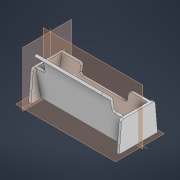
# Autodesk Inventor part: business card holder lgcc
Saved by Autodesk Inventor 2021 (Build 250183000, 183)
## iProperties
Created: 2020-08-19
Part Number: business card holder lgcc
Material: Generic
Document SubType Name: Modeling
Designer: brand
Density: 1 g/cm^3
Appearance: Default
Author: brand
Autodesk Inventor part; units mm, degrees
(part 1 of 6)
sketch "Block1" plane through (0, 0, 0) normal (0, 0, 1) x (1, 0, 0)
  line L0 (3.2262, -16.0033) -> (3.2322, -15.9973)
  spline S0 degree 3 poles (3.2322, -15.9973) (3.2262, -15.9973) (3.2262, -16.0033) (3.2262, -16.0033) knots 1 1 1 1 2 2 2 2
  line L1 (3.2322, -15.9973) -> (3.2262, -15.9973) construction
  line L2 (3.2262, -15.9973) -> (3.2262, -16.0033) construction
  line L3 (3.2262, -16.0033) -> (3.2262, -16.0033) construction
  line L4 (38.8954, -13.7894) -> (38.8894, -13.8014)
  spline S1 degree 3 poles (38.8894, -13.8014) (38.8895, -13.8014) (38.8954, -13.7954) (38.8954, -13.7894) knots 1 1 1 1 2 2 2 2
  line L5 (38.8894, -13.8014) -> (38.8894, -13.8014) construction
  line L6 (38.8894, -13.8014) -> (38.8954, -13.7954) construction
  line L7 (38.8954, -13.7954) -> (38.8954, -13.7894) construction
  spline S2 degree 3 poles (38.8894, -13.8014) (38.8835, -13.8074) (38.8774, -13.8134) (38.8774, -13.8194) knots 0 0 0 0 1 1 1 1
  line L8 (38.8894, -13.8014) -> (38.8835, -13.8074) construction
  line L9 (38.8835, -13.8074) -> (38.8774, -13.8134) construction
  line L10 (38.8774, -13.8134) -> (38.8774, -13.8194) construction
  spline S3 degree 3 poles (38.8774, -13.8194) (38.8774, -13.8194) (38.8835, -13.8134) (38.8894, -13.8014) knots 1 1 1 1 2 2 2 2
  line L11 (38.8774, -13.8194) -> (38.8774, -13.8194) construction
  line L12 (38.8774, -13.8194) -> (38.8835, -13.8134) construction
  line L13 (38.8835, -13.8134) -> (38.8894, -13.8014) construction
  spline S4 degree 3 poles (51.5732, -15.5233) (51.5732, -15.4813) (51.6092, -15.4273) (51.5732, -15.3793) (51.5432, -15.3433) (51.5432, -15.3673) (51.5132, -15.3613) (51.3932, -15.3133) (51.2792, -15.3433) (51.1712, -15.3973) (51.0332, -15.4693) (50.8112, -15.7153) (50.8952, -15.8953) (50.9192, -15.9433) (51.0272, -16.0393) (51.0692, -16.0573) (51.1832, -16.1173) (51.2432, -16.0393) (51.3152, -15.9733) (51.3992, -15.8953) (51.4592, -15.8653) (51.5012, -15.7693) (51.5132, -15.7453) (51.6572, -15.5233) (51.5732, -15.5233) knots 0 0 0 0 1 1 1 2 2 2 3 3 3 4 4 4 5 5 5 6 6 6 7 7 7 8 8 8 8
  line L14 (51.5732, -15.5233) -> (51.5732, -15.4813) construction
  line L15 (51.5732, -15.4813) -> (51.6092, -15.4273) construction
  line L16 (51.6092, -15.4273) -> (51.5732, -15.3793) construction
  line L17 (51.5732, -15.3793) -> (51.5432, -15.3433) construction
  line L18 (51.5432, -15.3433) -> (51.5432, -15.3673) construction
  line L19 (51.5432, -15.3673) -> (51.5132, -15.3613) construction
  line L20 (51.5132, -15.3613) -> (51.3932, -15.3133) construction
  line L21 (51.3932, -15.3133) -> (51.2792, -15.3433) construction
  line L22 (51.2792, -15.3433) -> (51.1712, -15.3973) construction
  line L23 (51.1712, -15.3973) -> (51.0332, -15.4693) construction
  line L24 (51.0332, -15.4693) -> (50.8112, -15.7153) construction
  line L25 (50.8112, -15.7153) -> (50.8952, -15.8953) construction
  line L26 (50.8952, -15.8953) -> (50.9192, -15.9433) construction
  line L27 (50.9192, -15.9433) -> (51.0272, -16.0393) construction
  line L28 (51.0272, -16.0393) -> (51.0692, -16.0573) construction
  line L29 (51.0692, -16.0573) -> (51.1832, -16.1173) construction
  line L30 (51.1832, -16.1173) -> (51.2432, -16.0393) construction
  line L31 (51.2432, -16.0393) -> (51.3152, -15.9733) construction
  line L32 (51.3152, -15.9733) -> (51.3992, -15.8953) construction
  line L33 (51.3992, -15.8953) -> (51.4592, -15.8653) construction
  line L34 (51.4592, -15.8653) -> (51.5012, -15.7693) construction
  line L35 (51.5012, -15.7693) -> (51.5132, -15.7453) construction
  line L36 (51.5132, -15.7453) -> (51.6572, -15.5233) construction
  line L37 (51.6572, -15.5233) -> (51.5732, -15.5233) construction
  spline S5 degree 3 poles (51.0512, -14.0894) (51.0512, -14.0894) (51.0572, -14.0954) (51.0512, -14.0834) knots 0 0 0 0 1 1 1 1
  line L38 (51.0512, -14.0894) -> (51.0512, -14.0894) construction
  line L39 (51.0512, -14.0894) -> (51.0572, -14.0954) construction
  line L40 (51.0572, -14.0954) -> (51.0512, -14.0834) construction
  spline S6 degree 3 poles (51.0512, -14.0834) (51.0212, -14.0414) (50.9792, -14.0714) (50.9372, -14.0834) knots 1 1 1 1 2 2 2 2
  line L41 (51.0512, -14.0834) -> (51.0212, -14.0414) construction
  line L42 (51.0212, -14.0414) -> (50.9792, -14.0714) construction
  line L43 (50.9792, -14.0714) -> (50.9372, -14.0834) construction
  spline S7 degree 3 poles (50.9372, -14.0834) (50.7632, -14.1194) (50.5832, -14.1614) (50.4032, -14.1914) knots 2 2 2 2 3 3 3 3
  line L44 (50.9372, -14.0834) -> (50.7632, -14.1194) construction
  line L45 (50.7632, -14.1194) -> (50.5832, -14.1614) construction
  line L46 (50.5832, -14.1614) -> (50.4032, -14.1914) construction
  spline S8 degree 3 poles (50.4032, -14.1914) (50.4692, -13.9754) (50.5352, -13.7474) (50.5592, -13.5254) knots 3 3 3 3 4 4 4 4
  line L47 (50.4032, -14.1914) -> (50.4692, -13.9754) construction
  line L48 (50.4692, -13.9754) -> (50.5352, -13.7474) construction
  line L49 (50.5352, -13.7474) -> (50.5592, -13.5254) construction
  spline S9 degree 3 poles (50.5592, -13.5254) (50.5712, -13.4414) (50.5772, -13.3514) (50.5592, -13.2674) knots 4 4 4 4 5 5 5 5
  line L50 (50.5592, -13.5254) -> (50.5712, -13.4414) construction
  line L51 (50.5712, -13.4414) -> (50.5772, -13.3514) construction
  line L52 (50.5772, -13.3514) -> (50.5592, -13.2674) construction
  spline S10 degree 3 poles (50.5592, -13.2674) (50.5472, -13.2134) (50.5292, -13.1594) (50.4992, -13.1114) knots 5 5 5 5 6 6 6 6
  line L53 (50.5592, -13.2674) -> (50.5472, -13.2134) construction
  line L54 (50.5472, -13.2134) -> (50.5292, -13.1594) construction
  line L55 (50.5292, -13.1594) -> (50.4992, -13.1114) construction
  spline S11 degree 3 poles (50.4992, -13.1114) (50.4992, -13.1113) (50.4272, -13.0214) (50.4452, -13.0694) knots 6 6 6 6 7 7 7 7
  line L56 (50.4992, -13.1114) -> (50.4992, -13.1114) construction
  line L57 (50.4992, -13.1114) -> (50.4272, -13.0214) construction
  line L58 (50.4272, -13.0214) -> (50.4452, -13.0694) construction
  line L59 (50.4452, -13.0694) -> (50.4392, -13.0634)
  line L60 (50.4392, -13.0634) -> (50.4152, -13.0154)
  line L61 (50.4152, -13.0154) -> (50.4392, -13.0394)
  spline S12 degree 3 poles (50.4392, -13.0394) (50.4452, -13.0034) (50.3433, -12.9374) (50.3432, -12.9374) knots 10 10 10 10 11 11 11 11
  line L62 (50.4392, -13.0394) -> (50.4452, -13.0034) construction
  line L63 (50.4452, -13.0034) -> (50.3432, -12.9374) construction
  line L64 (50.3432, -12.9374) -> (50.3432, -12.9374) construction
  spline S13 degree 3 poles (50.3432, -12.9374) (50.1932, -12.7874) (49.9892, -12.6734) (49.7852, -12.7874) knots 11 11 11 11 12 12 12 12
  line L65 (50.3432, -12.9374) -> (50.1932, -12.7874) construction
  line L66 (50.1932, -12.7874) -> (49.9892, -12.6734) construction
  line L67 (49.9892, -12.6734) -> (49.7852, -12.7874) construction
  spline S14 degree 3 poles (49.7852, -12.7874) (49.6592, -12.8594) (49.5573, -12.9794) (49.4732, -13.0994) knots 12 12 12 12 13 13 13 13
  line L68 (49.7852, -12.7874) -> (49.6592, -12.8594) construction
  line L69 (49.6592, -12.8594) -> (49.5573, -12.9794) construction
  line L70 (49.5573, -12.9794) -> (49.4732, -13.0994) construction
  spline S15 degree 3 poles (49.4732, -13.0994) (49.4432, -13.1414) (49.4132, -13.1894) (49.3892, -13.2374) knots 13 13 13 13 14 14 14 14
  line L71 (49.4732, -13.0994) -> (49.4432, -13.1414) construction
  line L72 (49.4432, -13.1414) -> (49.4132, -13.1894) construction
  line L73 (49.4132, -13.1894) -> (49.3892, -13.2374) construction
  spline S16 degree 3 poles (49.3892, -13.2374) (49.3652, -13.2854) (49.3292, -13.4414) (49.2933, -13.4654) knots 14 14 14 14 15 15 15 15
  line L74 (49.3892, -13.2374) -> (49.3652, -13.2854) construction
  line L75 (49.3652, -13.2854) -> (49.3292, -13.4414) construction
  line L76 (49.3292, -13.4414) -> (49.2933, -13.4654) construction
  spline S17 degree 3 poles (49.2933, -13.4654) (49.2632, -13.4894) (49.1733, -13.4954) (49.1312, -13.5194) knots 15 15 15 15 16 16 16 16
  line L77 (49.2933, -13.4654) -> (49.2632, -13.4894) construction
  line L78 (49.2632, -13.4894) -> (49.1733, -13.4954) construction
  line L79 (49.1733, -13.4954) -> (49.1312, -13.5194) construction
  spline S18 degree 3 poles (49.1312, -13.5194) (49.0712, -13.5434) (49.0173, -13.5734) (48.9692, -13.6094) knots 16 16 16 16 17 17 17 17
  line L80 (49.1312, -13.5194) -> (49.0712, -13.5434) construction
  line L81 (49.0712, -13.5434) -> (49.0173, -13.5734) construction
  line L82 (49.0173, -13.5734) -> (48.9692, -13.6094) construction
  spline S19 degree 3 poles (48.9692, -13.6094) (48.8553, -13.6814) (48.7653, -13.7834) (48.6812, -13.8854) knots 17 17 17 17 18 18 18 18
  line L83 (48.9692, -13.6094) -> (48.8553, -13.6814) construction
  line L84 (48.8553, -13.6814) -> (48.7653, -13.7834) construction
  line L85 (48.7653, -13.7834) -> (48.6812, -13.8854) construction
  spline S20 degree 3 poles (48.6812, -13.8854) (48.5373, -14.0774) (48.4653, -14.2934) (48.3632, -14.4854) knots 18 18 18 18 19 19 19 19
  line L86 (48.6812, -13.8854) -> (48.5373, -14.0774) construction
  line L87 (48.5373, -14.0774) -> (48.4653, -14.2934) construction
  line L88 (48.4653, -14.2934) -> (48.3632, -14.4854) construction
  spline S21 degree 3 poles (48.3632, -14.4854) (48.1713, -14.8513) (48.3813, -15.3313) (48.7353, -15.5053) knots 19 19 19 19 20 20 20 20
  line L89 (48.3632, -14.4854) -> (48.1713, -14.8513) construction
  line L90 (48.1713, -14.8513) -> (48.3813, -15.3313) construction
  line L91 (48.3813, -15.3313) -> (48.7353, -15.5053) construction
  spline S22 degree 3 poles (48.7353, -15.5053) (48.8492, -15.5593) (48.9812, -15.5833) (49.1012, -15.5713) knots 20 20 20 20 21 21 21 21
  line L92 (48.7353, -15.5053) -> (48.8492, -15.5593) construction
  line L93 (48.8492, -15.5593) -> (48.9812, -15.5833) construction
  line L94 (48.9812, -15.5833) -> (49.1012, -15.5713) construction
  spline S23 degree 3 poles (49.1012, -15.5713) (49.2273, -15.5533) (49.3472, -15.4873) (49.4432, -15.4153) knots 21 21 21 21 22 22 22 22
  line L95 (49.1012, -15.5713) -> (49.2273, -15.5533) construction
  line L96 (49.2273, -15.5533) -> (49.3472, -15.4873) construction
  line L97 (49.3472, -15.4873) -> (49.4432, -15.4153) construction
  spline S24 degree 3 poles (49.4432, -15.4153) (49.5332, -15.3493) (49.7312, -15.2293) (49.7672, -15.1273) knots 22 22 22 22 23 23 23 23
  line L98 (49.4432, -15.4153) -> (49.5332, -15.3493) construction
  line L99 (49.5332, -15.3493) -> (49.7312, -15.2293) construction
  line L100 (49.7312, -15.2293) -> (49.7672, -15.1273) construction
  spline S25 degree 3 poles (49.7672, -15.1273) (49.7672, -15.1213) (49.7552, -15.1273) (49.7372, -15.1453) knots 23 23 23 23 24 24 24 24
  line L101 (49.7672, -15.1273) -> (49.7672, -15.1213) construction
  line L102 (49.7672, -15.1213) -> (49.7552, -15.1273) construction
  line L103 (49.7552, -15.1273) -> (49.7372, -15.1453) construction
  line L104 (49.7372, -15.1453) -> (49.9112, -14.9413)
  spline S26 degree 3 poles (49.9112, -14.9413) (49.9172, -14.9473) (49.8693, -15.0073) (49.8692, -15.0073) knots 25 25 25 25 26 26 26 26
  line L105 (49.9112, -14.9413) -> (49.9172, -14.9473) construction
  line L106 (49.9172, -14.9473) -> (49.8692, -15.0073) construction
  line L107 (49.8692, -15.0073) -> (49.8692, -15.0073) construction
  spline S27 degree 3 poles (49.8692, -15.0073) (49.9112, -15.0253) (50.1272, -14.7074) (50.1512, -14.6833) knots 26 26 26 26 27 27 27 27
  line L108 (49.8692, -15.0073) -> (49.9112, -15.0253) construction
  line L109 (49.9112, -15.0253) -> (50.1272, -14.7074) construction
  line L110 (50.1272, -14.7074) -> (50.1512, -14.6833) construction
  spline S28 degree 3 poles (50.1512, -14.6833) (50.1932, -14.6113) (50.2352, -14.5333) (50.2832, -14.4614) knots 27 27 27 27 28 28 28 28
  line L111 (50.1512, -14.6833) -> (50.1932, -14.6113) construction
  line L112 (50.1932, -14.6113) -> (50.2352, -14.5333) construction
  line L113 (50.2352, -14.5333) -> (50.2832, -14.4614) construction
  spline S29 degree 3 poles (50.2832, -14.4614) (50.3252, -14.4073) (50.3132, -14.4134) (50.3732, -14.3894) knots 28 28 28 28 29 29 29 29
  line L114 (50.2832, -14.4614) -> (50.3252, -14.4073) construction
  line L115 (50.3252, -14.4073) -> (50.3132, -14.4134) construction
  line L116 (50.3132, -14.4134) -> (50.3732, -14.3894) construction
  spline S30 degree 3 poles (50.3732, -14.3894) (50.3672, -14.3954) (50.4452, -14.3714) (50.4572, -14.3714) knots 29 29 29 29 30 30 30 30
  line L117 (50.3732, -14.3894) -> (50.3672, -14.3954) construction
  line L118 (50.3672, -14.3954) -> (50.4452, -14.3714) construction
  line L119 (50.4452, -14.3714) -> (50.4572, -14.3714) construction
  spline S31 degree 3 poles (50.4572, -14.3714) (50.5232, -14.3594) (51.2252, -14.3114) (51.0512, -14.0894) knots 30 30 30 30 31 31 31 31
  line L120 (50.4572, -14.3714) -> (50.5232, -14.3594) construction
  line L121 (50.5232, -14.3594) -> (51.2252, -14.3114) construction
  line L122 (51.2252, -14.3114) -> (51.0512, -14.0894) construction
  spline S32 degree 3 poles (49.7492, -13.2434) (49.7492, -13.2494) (49.7433, -13.2494) (49.7432, -13.2494) knots 0 0 0 0 1 1 1 1
  line L123 (49.7492, -13.2434) -> (49.7492, -13.2494) construction
  line L124 (49.7492, -13.2494) -> (49.7432, -13.2494) construction
  line L125 (49.7432, -13.2494) -> (49.7432, -13.2494) construction
  line L126 (49.7432, -13.2494) -> (49.7492, -13.2434)
  line L127 (49.7492, -13.2434) -> (49.7432, -13.2494)
  spline S33 degree 3 poles (49.7432, -13.2494) (49.7433, -13.2494) (49.7492, -13.2494) (49.7492, -13.2434) knots 1 1 1 1 2 2 2 2
  line L128 (49.7432, -13.2494) -> (49.7432, -13.2494) construction
  line L129 (49.7432, -13.2494) -> (49.7492, -13.2494) construction
  line L130 (49.7492, -13.2494) -> (49.7492, -13.2434) construction
  spline S34 degree 3 poles (47.9672, -14.3534) (47.9012, -14.3474) (47.8532, -14.4914) (47.8292, -14.5273) knots 0 0 0 0 1 1 1 1
  line L131 (47.9672, -14.3534) -> (47.9012, -14.3474) construction
  line L132 (47.9012, -14.3474) -> (47.8532, -14.4914) construction
  line L133 (47.8532, -14.4914) -> (47.8292, -14.5273) construction
  spline S35 degree 3 poles (47.8292, -14.5273) (47.6493, -14.8214) (47.4392, -15.0974) (47.2052, -15.3493) knots 1 1 1 1 2 2 2 2
  line L134 (47.8292, -14.5273) -> (47.6493, -14.8214) construction
  line L135 (47.6493, -14.8214) -> (47.4392, -15.0974) construction
  line L136 (47.4392, -15.0974) -> (47.2052, -15.3493) construction
  spline S36 degree 3 poles (47.2052, -15.3493) (46.9653, -15.6133) (46.6652, -15.8953) (46.2993, -15.9793) knots 2 2 2 2 3 3 3 3
  line L137 (47.2052, -15.3493) -> (46.9653, -15.6133) construction
  line L138 (46.9653, -15.6133) -> (46.6652, -15.8953) construction
  line L139 (46.6652, -15.8953) -> (46.2993, -15.9793) construction
  spline S37 degree 3 poles (46.2993, -15.9793) (46.2513, -15.9913) (46.1973, -15.9973) (46.1433, -15.9973) knots 3 3 3 3 4 4 4 4
  line L140 (46.2993, -15.9793) -> (46.2513, -15.9913) construction
  line L141 (46.2513, -15.9913) -> (46.1973, -15.9973) construction
  line L142 (46.1973, -15.9973) -> (46.1433, -15.9973) construction
  spline S38 degree 3 poles (46.1433, -15.9973) (46.0712, -15.9913) (46.0052, -15.9733) (45.9513, -15.9193) knots 4 4 4 4 5 5 5 5
  line L143 (46.1433, -15.9973) -> (46.0712, -15.9913) construction
  line L144 (46.0712, -15.9913) -> (46.0052, -15.9733) construction
  line L145 (46.0052, -15.9733) -> (45.9513, -15.9193) construction
  spline S39 degree 3 poles (45.9513, -15.9193) (45.9213, -15.8893) (45.8913, -15.7873) (45.8553, -15.7693) knots 5 5 5 5 6 6 6 6
  line L146 (45.9513, -15.9193) -> (45.9213, -15.8893) construction
  line L147 (45.9213, -15.8893) -> (45.8913, -15.7873) construction
  line L148 (45.8913, -15.7873) -> (45.8553, -15.7693) construction
  spline S40 degree 3 poles (45.8553, -15.7693) (45.8553, -15.7393) (45.8493, -15.7093) (45.8433, -15.6913) knots 6 6 6 6 7 7 7 7
  line L149 (45.8553, -15.7693) -> (45.8553, -15.7393) construction
  line L150 (45.8553, -15.7393) -> (45.8493, -15.7093) construction
  line L151 (45.8493, -15.7093) -> (45.8433, -15.6913) construction
  line L152 (45.8433, -15.6913) -> (45.8351, -15.6553)
  spline S41 degree 3 poles (45.8351, -15.6553) (45.8291, -15.4753) (45.8333, -15.3073) (45.875, -15.1213) knots 8 8 8 8 9 9 9 9
  line L153 (45.8351, -15.6553) -> (45.8291, -15.4753) construction
  line L154 (45.8291, -15.4753) -> (45.8333, -15.3073) construction
  line L155 (45.8333, -15.3073) -> (45.875, -15.1213) construction
  line L156 (45.875, -15.1213) -> (45.875, -15.1153)
  spline S42 degree 3 poles (45.875, -15.1153) (45.875, -15.1101) (45.8724, -15.1089) (45.8717, -15.1049) knots 10 10 10 10 11 11 11 11
  line L157 (45.875, -15.1153) -> (45.875, -15.1101) construction
  line L158 (45.875, -15.1101) -> (45.8724, -15.1089) construction
  line L159 (45.8724, -15.1089) -> (45.8717, -15.1049) construction
  spline S43 degree 3 poles (45.8717, -15.1049) (45.8737, -15.1029) (45.875, -15.1011) (45.875, -15.0974) knots 11 11 11 11 12 12 12 12
  line L160 (45.8717, -15.1049) -> (45.8737, -15.1029) construction
  line L161 (45.8737, -15.1029) -> (45.875, -15.1011) construction
  line L162 (45.875, -15.1011) -> (45.875, -15.0974) construction
  line L163 (45.875, -15.0974) -> (45.875, -15.0673)
  spline S44 degree 3 poles (45.875, -15.0673) (45.9167, -14.7134) (46.0601, -14.3654) (46.1861, -14.0234) knots 13 13 13 13 14 14 14 14
  line L164 (45.875, -15.0673) -> (45.9167, -14.7134) construction
  line L165 (45.9167, -14.7134) -> (46.0601, -14.3654) construction
  line L166 (46.0601, -14.3654) -> (46.1861, -14.0234) construction
  spline S45 degree 3 poles (46.1861, -14.0234) (46.3181, -13.6634) (46.4407, -13.3094) (46.6087, -12.9674) knots 14 14 14 14 15 15 15 15
  line L167 (46.1861, -14.0234) -> (46.3181, -13.6634) construction
  line L168 (46.3181, -13.6634) -> (46.4407, -13.3094) construction
  line L169 (46.4407, -13.3094) -> (46.6087, -12.9674) construction
  spline S46 degree 3 poles (46.6087, -12.9674) (46.7647, -12.6434) (46.943, -12.3254) (47.147, -12.0314) knots 15 15 15 15 16 16 16 16
  line L170 (46.6087, -12.9674) -> (46.7647, -12.6434) construction
  line L171 (46.7647, -12.6434) -> (46.943, -12.3254) construction
  line L172 (46.943, -12.3254) -> (47.147, -12.0314) construction
  spline S47 degree 3 poles (47.147, -12.0314) (47.3269, -11.7614) (47.5421, -11.4674) (47.8181, -11.2874) knots 16 16 16 16 17 17 17 17
  line L173 (47.147, -12.0314) -> (47.3269, -11.7614) construction
  line L174 (47.3269, -11.7614) -> (47.5421, -11.4674) construction
  line L175 (47.5421, -11.4674) -> (47.8181, -11.2874) construction
  spline S48 degree 3 poles (47.8181, -11.2874) (47.9021, -11.2634) (47.9857, -11.1734) (48.0937, -11.1914) knots 17 17 17 17 18 18 18 18
  line L176 (47.8181, -11.2874) -> (47.9021, -11.2634) construction
  line L177 (47.9021, -11.2634) -> (47.9857, -11.1734) construction
  line L178 (47.9857, -11.1734) -> (48.0937, -11.1914) construction
  spline S49 degree 3 poles (48.0937, -11.1914) (48.2017, -11.2094) (48.2014, -11.3234) (48.1774, -11.4314) knots 18 18 18 18 19 19 19 19
  line L179 (48.0937, -11.1914) -> (48.2017, -11.2094) construction
  line L180 (48.2017, -11.2094) -> (48.2014, -11.3234) construction
  line L181 (48.2014, -11.3234) -> (48.1774, -11.4314) construction
  spline S50 degree 3 poles (48.1774, -11.4314) (48.2074, -11.3474) (48.2253, -11.2574) (48.1534, -11.1974) knots 19 19 19 19 20 20 20 20
  line L182 (48.1774, -11.4314) -> (48.2074, -11.3474) construction
  line L183 (48.2074, -11.3474) -> (48.2253, -11.2574) construction
  line L184 (48.2253, -11.2574) -> (48.1534, -11.1974) construction
  spline S51 degree 3 poles (48.1534, -11.1974) (48.0573, -11.1254) (47.8713, -11.2394) (47.7933, -11.2934) knots 20 20 20 20 21 21 21 21
  line L185 (48.1534, -11.1974) -> (48.0573, -11.1254) construction
  line L186 (48.0573, -11.1254) -> (47.8713, -11.2394) construction
  line L187 (47.8713, -11.2394) -> (47.7933, -11.2934) construction
  spline S52 degree 3 poles (47.7933, -11.2934) (47.7573, -11.3054) (47.7213, -11.3294) (47.6913, -11.3534) knots 21 21 21 21 22 22 22 22
  line L188 (47.7933, -11.2934) -> (47.7573, -11.3054) construction
  line L189 (47.7573, -11.3054) -> (47.7213, -11.3294) construction
  line L190 (47.7213, -11.3294) -> (47.6913, -11.3534) construction
  spline S53 degree 3 poles (47.6913, -11.3534) (47.7093, -11.3354) (47.7332, -11.3174) (47.7632, -11.2994) knots 22 22 22 22 23 23 23 23
  line L191 (47.6913, -11.3534) -> (47.7093, -11.3354) construction
  line L192 (47.7093, -11.3354) -> (47.7332, -11.3174) construction
  line L193 (47.7332, -11.3174) -> (47.7632, -11.2994) construction
  line L194 (47.7632, -11.2994) -> (47.7332, -11.3114)
  line L195 (47.7332, -11.3114) -> (47.8172, -11.2634)
  spline S54 degree 3 poles (47.8172, -11.2634) (47.9132, -11.2094) (48.1292, -11.0894) (48.2012, -11.2454) knots 25 25 25 25 26 26 26 26
  line L196 (47.8172, -11.2634) -> (47.9132, -11.2094) construction
  line L197 (47.9132, -11.2094) -> (48.1292, -11.0894) construction
  line L198 (48.1292, -11.0894) -> (48.2012, -11.2454) construction
  spline S55 degree 3 poles (48.2012, -11.2454) (48.2552, -11.3714) (48.1712, -11.5814) (48.1292, -11.7014) knots 26 26 26 26 27 27 27 27
  line L199 (48.2012, -11.2454) -> (48.2552, -11.3714) construction
  line L200 (48.2552, -11.3714) -> (48.1712, -11.5814) construction
  line L201 (48.1712, -11.5814) -> (48.1292, -11.7014) construction
  spline S56 degree 3 poles (48.1292, -11.7014) (48.0512, -11.9054) (47.9552, -12.0974) (47.8532, -12.2894) knots 27 27 27 27 28 28 28 28
  line L202 (48.1292, -11.7014) -> (48.0512, -11.9054) construction
  line L203 (48.0512, -11.9054) -> (47.9552, -12.0974) construction
  line L204 (47.9552, -12.0974) -> (47.8532, -12.2894) construction
  spline S57 degree 3 poles (47.8532, -12.2894) (47.8712, -12.2474) (47.9432, -12.0887) (47.9432, -12.0885) knots 28 28 28 28 29 29 29 29
  line L205 (47.8532, -12.2894) -> (47.8712, -12.2474) construction
  line L206 (47.8712, -12.2474) -> (47.9432, -12.0885) construction
  line L207 (47.9432, -12.0885) -> (47.9432, -12.0885) construction
  spline S58 degree 3 poles (47.9432, -12.0885) (47.9012, -12.0825) (47.7092, -12.5417) (47.6732, -12.5417) knots 29 29 29 29 30 30 30 30
  line L208 (47.9432, -12.0885) -> (47.9012, -12.0825) construction
  line L209 (47.9012, -12.0825) -> (47.7092, -12.5417) construction
  line L210 (47.7092, -12.5417) -> (47.6732, -12.5417) construction
  line L211 (47.6732, -12.5417) -> (47.6792, -12.5417)
  spline S59 degree 3 poles (47.6792, -12.5417) (47.6552, -12.5417) (47.6372, -12.5745) (47.6372, -12.5805) knots 31 31 31 31 32 32 32 32
  line L212 (47.6792, -12.5417) -> (47.6552, -12.5417) construction
  line L213 (47.6552, -12.5417) -> (47.6372, -12.5745) construction
  line L214 (47.6372, -12.5745) -> (47.6372, -12.5805) construction
  spline S60 degree 3 poles (47.6372, -12.5805) (47.6252, -12.6525) (47.7092, -12.633) (47.7572, -12.627) knots 32 32 32 32 33 33 33 33
  line L215 (47.6372, -12.5805) -> (47.6252, -12.6525) construction
  line L216 (47.6252, -12.6525) -> (47.7092, -12.633) construction
  line L217 (47.7092, -12.633) -> (47.7572, -12.627) construction
  spline S61 degree 3 poles (47.7572, -12.627) (47.9612, -12.603) (48.2184, -12.4282) (48.3504, -12.2782) knots 33 33 33 33 34 34 34 34
  line L218 (47.7572, -12.627) -> (47.9612, -12.603) construction
  line L219 (47.9612, -12.603) -> (48.2184, -12.4282) construction
  line L220 (48.2184, -12.4282) -> (48.3504, -12.2782) construction
  spline S62 degree 3 poles (48.3504, -12.2782) (48.4945, -12.1162) (48.5417, -11.8694) (48.5417, -11.6534) knots 34 34 34 34 35 35 35 35
  line L221 (48.3504, -12.2782) -> (48.4945, -12.1162) construction
  line L222 (48.4945, -12.1162) -> (48.5417, -11.8694) construction
  line L223 (48.5417, -11.8694) -> (48.5417, -11.6534) construction
  line L224 (48.5417, -11.6534) -> (48.5417, -11.6474)
  spline S63 degree 3 poles (48.5417, -11.6474) (48.5417, -11.2394) (48.2604, -10.7234) (47.7745, -10.7534) knots 36 36 36 36 37 37 37 37
  line L225 (48.5417, -11.6474) -> (48.5417, -11.2394) construction
  line L226 (48.5417, -11.2394) -> (48.2604, -10.7234) construction
  line L227 (48.2604, -10.7234) -> (47.7745, -10.7534) construction
  spline S64 degree 3 poles (47.7745, -10.7534) (47.5045, -10.7654) (47.2559, -11.0294) (47.0819, -11.2094) knots 37 37 37 37 38 38 38 38
  line L228 (47.7745, -10.7534) -> (47.5045, -10.7654) construction
  line L229 (47.5045, -10.7654) -> (47.2559, -11.0294) construction
  line L230 (47.2559, -11.0294) -> (47.0819, -11.2094) construction
  spline S65 degree 3 poles (47.0819, -11.2094) (46.9559, -11.3534) (46.8375, -11.5094) (46.7295, -11.6654) knots 38 38 38 38 39 39 39 39
  line L231 (47.0819, -11.2094) -> (46.9559, -11.3534) construction
  line L232 (46.9559, -11.3534) -> (46.8375, -11.5094) construction
  line L233 (46.8375, -11.5094) -> (46.7295, -11.6654) construction
  spline S66 degree 3 poles (46.7295, -11.6654) (46.6816, -11.7374) (46.6344, -11.8034) (46.5924, -11.8754) knots 39 39 39 39 40 40 40 40
  line L234 (46.7295, -11.6654) -> (46.6816, -11.7374) construction
  line L235 (46.6816, -11.7374) -> (46.6344, -11.8034) construction
  line L236 (46.6344, -11.8034) -> (46.5924, -11.8754) construction
  spline S67 degree 3 poles (46.5924, -11.8754) (46.5444, -11.9414) (46.4489, -12.0434) (46.4248, -12.1214) knots 40 40 40 40 41 41 41 41
  line L237 (46.5924, -11.8754) -> (46.5444, -11.9414) construction
  line L238 (46.5444, -11.9414) -> (46.4489, -12.0434) construction
  line L239 (46.4489, -12.0434) -> (46.4248, -12.1214) construction
  spline S68 degree 3 poles (46.4248, -12.1214) (46.4249, -12.1214) (46.455, -12.0854) (46.479, -12.0614) knots 41 41 41 41 42 42 42 42
  line L240 (46.4248, -12.1214) -> (46.4248, -12.1214) construction
  line L241 (46.4248, -12.1214) -> (46.455, -12.0854) construction
  line L242 (46.455, -12.0854) -> (46.479, -12.0614) construction
  spline S69 degree 3 poles (46.479, -12.0614) (46.413, -12.1634) (46.3531, -12.2714) (46.2931, -12.3734) knots 42 42 42 42 43 43 43 43
  line L243 (46.479, -12.0614) -> (46.413, -12.1634) construction
  line L244 (46.413, -12.1634) -> (46.3531, -12.2714) construction
  line L245 (46.3531, -12.2714) -> (46.2931, -12.3734) construction
  spline S70 degree 3 poles (46.2931, -12.3734) (46.2872, -12.3674) (46.3292, -12.2835) (46.3292, -12.2834) knots 43 43 43 43 44 44 44 44
  line L246 (46.2931, -12.3734) -> (46.2872, -12.3674) construction
  line L247 (46.2872, -12.3674) -> (46.3292, -12.2834) construction
  line L248 (46.3292, -12.2834) -> (46.3292, -12.2834) construction
  spline S71 degree 3 poles (46.3292, -12.2834) (46.2752, -12.2714) (46.0292, -12.7634) (45.9992, -12.8174) knots 44 44 44 44 45 45 45 45
  line L249 (46.3292, -12.2834) -> (46.2752, -12.2714) construction
  line L250 (46.2752, -12.2714) -> (46.0292, -12.7634) construction
  line L251 (46.0292, -12.7634) -> (45.9992, -12.8174) construction
  spline S72 degree 3 poles (45.9992, -12.8174) (45.8912, -13.0154) (45.7953, -13.2134) (45.7293, -13.4234) knots 45 45 45 45 46 46 46 46
  line L252 (45.9992, -12.8174) -> (45.8912, -13.0154) construction
  line L253 (45.8912, -13.0154) -> (45.7953, -13.2134) construction
  line L254 (45.7953, -13.2134) -> (45.7293, -13.4234) construction
  spline S73 degree 3 poles (45.7293, -13.4234) (45.6573, -13.6574) (45.5613, -13.8794) (45.4893, -14.1074) knots 46 46 46 46 47 47 47 47
  line L255 (45.7293, -13.4234) -> (45.6573, -13.6574) construction
  line L256 (45.6573, -13.6574) -> (45.5613, -13.8794) construction
  line L257 (45.5613, -13.8794) -> (45.4893, -14.1074) construction
  spline S74 degree 3 poles (45.4893, -14.1074) (45.4533, -14.2214) (45.4173, -14.3294) (45.3933, -14.4434) knots 47 47 47 47 48 48 48 48
  line L258 (45.4893, -14.1074) -> (45.4533, -14.2214) construction
  line L259 (45.4533, -14.2214) -> (45.4173, -14.3294) construction
  line L260 (45.4173, -14.3294) -> (45.3933, -14.4434) construction
  spline S75 degree 3 poles (45.3933, -14.4434) (45.3813, -14.4974) (45.3693, -14.5453) (45.3633, -14.5993) knots 48 48 48 48 49 49 49 49
  line L261 (45.3933, -14.4434) -> (45.3813, -14.4974) construction
  line L262 (45.3813, -14.4974) -> (45.3693, -14.5453) construction
  line L263 (45.3693, -14.5453) -> (45.3633, -14.5993) construction
  spline S76 degree 3 poles (45.3633, -14.5993) (45.3633, -14.6053) (45.3513, -14.7014) (45.3633, -14.6894) knots 49 49 49 49 50 50 50 50
  line L264 (45.3633, -14.5993) -> (45.3633, -14.6053) construction
  line L265 (45.3633, -14.6053) -> (45.3513, -14.7014) construction
  line L266 (45.3513, -14.7014) -> (45.3633, -14.6894) construction
  spline S77 degree 3 poles (45.3633, -14.6894) (45.3513, -14.7313) (45.3513, -14.7853) (45.3453, -14.8274) knots 50 50 50 50 51 51 51 51
  line L267 (45.3633, -14.6894) -> (45.3513, -14.7313) construction
  line L268 (45.3513, -14.7313) -> (45.3513, -14.7853) construction
  line L269 (45.3513, -14.7853) -> (45.3453, -14.8274) construction
  spline S78 degree 3 poles (45.3453, -14.8274) (45.3453, -14.8272) (45.3453, -14.7253) (45.3513, -14.7134) knots 51 51 51 51 52 52 52 52
  line L270 (45.3453, -14.8274) -> (45.3453, -14.8274) construction
  line L271 (45.3453, -14.8274) -> (45.3453, -14.7253) construction
  line L272 (45.3453, -14.7253) -> (45.3513, -14.7134) construction
  spline S79 degree 3 poles (45.3513, -14.7134) (45.3273, -14.7433) (45.3453, -14.8573) (45.3393, -14.8693) knots 52 52 52 52 53 53 53 53
  line L273 (45.3513, -14.7134) -> (45.3273, -14.7433) construction
  line L274 (45.3273, -14.7433) -> (45.3453, -14.8573) construction
  line L275 (45.3453, -14.8573) -> (45.3393, -14.8693) construction
  spline S80 degree 3 poles (45.3393, -14.8693) (45.3093, -15.0974) (45.2613, -15.3373) (45.3393, -15.5593) knots 53 53 53 53 54 54 54 54
  line L276 (45.3393, -14.8693) -> (45.3093, -15.0974) construction
  line L277 (45.3093, -15.0974) -> (45.2613, -15.3373) construction
  line L278 (45.2613, -15.3373) -> (45.3393, -15.5593) construction
  spline S81 degree 3 poles (45.3393, -15.5593) (45.4413, -15.8653) (45.6933, -16.1173) (45.9693, -16.2793) knots 54 54 54 54 55 55 55 55
  line L279 (45.3393, -15.5593) -> (45.4413, -15.8653) construction
  line L280 (45.4413, -15.8653) -> (45.6933, -16.1173) construction
  line L281 (45.6933, -16.1173) -> (45.9693, -16.2793) construction
  spline S82 degree 3 poles (45.9693, -16.2793) (46.1133, -16.3693) (46.3053, -16.4713) (46.4853, -16.4593) knots 55 55 55 55 56 56 56 56
  line L282 (45.9693, -16.2793) -> (46.1133, -16.3693) construction
  line L283 (46.1133, -16.3693) -> (46.3053, -16.4713) construction
  line L284 (46.3053, -16.4713) -> (46.4853, -16.4593) construction
  spline S83 degree 3 poles (46.4853, -16.4593) (46.6953, -16.4473) (46.8993, -16.2733) (47.0553, -16.1473) knots 56 56 56 56 57 57 57 57
  line L285 (46.4853, -16.4593) -> (46.6953, -16.4473) construction
  line L286 (46.6953, -16.4473) -> (46.8993, -16.2733) construction
  line L287 (46.8993, -16.2733) -> (47.0553, -16.1473) construction
  spline S84 degree 3 poles (47.0553, -16.1473) (47.5112, -15.7633) (47.9252, -15.2233) (48.0032, -14.6113) knots 57 57 57 57 58 58 58 58
  line L288 (47.0553, -16.1473) -> (47.5112, -15.7633) construction
  line L289 (47.5112, -15.7633) -> (47.9252, -15.2233) construction
  line L290 (47.9252, -15.2233) -> (48.0032, -14.6113) construction
  spline S85 degree 3 poles (48.0032, -14.6113) (48.0092, -14.5694) (48.0392, -14.3594) (47.9672, -14.3534) knots 58 58 58 58 59 59 59 59
  line L291 (48.0032, -14.6113) -> (48.0092, -14.5694) construction
  line L292 (48.0092, -14.5694) -> (48.0392, -14.3594) construction
  line L293 (48.0392, -14.3594) -> (47.9672, -14.3534) construction
  spline S86 degree 3 poles (48.1412, -11.5814) (48.1472, -11.5694) (48.1472, -11.5634) (48.1472, -11.5574) (48.1592, -11.5214) (48.1712, -11.4794) (48.1772, -11.4314) (48.1652, -11.4854) (48.1412, -11.5394) (48.1412, -11.5814) knots 0 0 0 0 1 1 1 2 2 2 3 3 3 3
  line L294 (48.1412, -11.5814) -> (48.1472, -11.5694) construction
  line L295 (48.1472, -11.5694) -> (48.1472, -11.5634) construction
  line L296 (48.1472, -11.5634) -> (48.1472, -11.5574) construction
  line L297 (48.1472, -11.5574) -> (48.1592, -11.5214) construction
  line L298 (48.1592, -11.5214) -> (48.1712, -11.4794) construction
  line L299 (48.1712, -11.4794) -> (48.1772, -11.4314) construction
  line L300 (48.1772, -11.4314) -> (48.1652, -11.4854) construction
  line L301 (48.1652, -11.4854) -> (48.1412, -11.5394) construction
  line L302 (48.1412, -11.5394) -> (48.1412, -11.5814) construction
  line L303 (44.0417, -14.0833) -> (44.0417, -14.0954)
  spline S87 degree 3 poles (44.0417, -14.0954) (43.9583, -13.9334) (43.8205, -14.1554) (43.7665, -14.2334) knots 1 1 1 1 2 2 2 2
  line L304 (44.0417, -14.0954) -> (43.9583, -13.9334) construction
  line L305 (43.9583, -13.9334) -> (43.8205, -14.1554) construction
  line L306 (43.8205, -14.1554) -> (43.7665, -14.2334) construction
  spline S88 degree 3 poles (43.7665, -14.2334) (43.6646, -14.3714) (43.5689, -14.5034) (43.4609, -14.6294) knots 2 2 2 2 3 3 3 3
  line L307 (43.7665, -14.2334) -> (43.6646, -14.3714) construction
  line L308 (43.6646, -14.3714) -> (43.5689, -14.5034) construction
  line L309 (43.5689, -14.5034) -> (43.4609, -14.6294) construction
  spline S89 degree 3 poles (43.4609, -14.6294) (43.3709, -14.7373) (43.2751, -14.8454) (43.2032, -14.9594) knots 3 3 3 3 4 4 4 4
  line L310 (43.4609, -14.6294) -> (43.3709, -14.7373) construction
  line L311 (43.3709, -14.7373) -> (43.2751, -14.8454) construction
  line L312 (43.2751, -14.8454) -> (43.2032, -14.9594) construction
  spline S90 degree 3 poles (43.2032, -14.9594) (43.2032, -14.9714) (43.1913, -15.0013) (43.1912, -15.0013) knots 4 4 4 4 5 5 5 5
  line L313 (43.2032, -14.9594) -> (43.2032, -14.9714) construction
  line L314 (43.2032, -14.9714) -> (43.1912, -15.0013) construction
  line L315 (43.1912, -15.0013) -> (43.1912, -15.0013) construction
  spline S91 degree 3 poles (43.1912, -15.0013) (43.1672, -15.0374) (43.1313, -15.0673) (43.1013, -15.1034) knots 5 5 5 5 6 6 6 6
  line L316 (43.1912, -15.0013) -> (43.1672, -15.0374) construction
  line L317 (43.1672, -15.0374) -> (43.1313, -15.0673) construction
  line L318 (43.1313, -15.0673) -> (43.1013, -15.1034) construction
  spline S92 degree 3 poles (43.1013, -15.1034) (43.0473, -15.1573) (42.9933, -15.2173) (42.9333, -15.2713) knots 6 6 6 6 7 7 7 7
  line L319 (43.1013, -15.1034) -> (43.0473, -15.1573) construction
  line L320 (43.0473, -15.1573) -> (42.9933, -15.2173) construction
  line L321 (42.9933, -15.2173) -> (42.9333, -15.2713) construction
  spline S93 degree 3 poles (42.9333, -15.2713) (42.8433, -15.3553) (42.3394, -15.8293) (42.2734, -15.5233) knots 7 7 7 7 8 8 8 8
  line L322 (42.9333, -15.2713) -> (42.8433, -15.3553) construction
  line L323 (42.8433, -15.3553) -> (42.3394, -15.8293) construction
  line L324 (42.3394, -15.8293) -> (42.2734, -15.5233) construction
  spline S94 degree 3 poles (42.2734, -15.5233) (42.2374, -15.3733) (42.2854, -15.1873) (42.3154, -15.0433) knots 8 8 8 8 9 9 9 9
  line L325 (42.2734, -15.5233) -> (42.2374, -15.3733) construction
  line L326 (42.2374, -15.3733) -> (42.2854, -15.1873) construction
  line L327 (42.2854, -15.1873) -> (42.3154, -15.0433) construction
  spline S95 degree 3 poles (42.3154, -15.0433) (42.3334, -14.9654) (42.3514, -14.8934) (42.3634, -14.8153) knots 9 9 9 9 10 10 10 10
  line L328 (42.3154, -15.0433) -> (42.3334, -14.9654) construction
  line L329 (42.3334, -14.9654) -> (42.3514, -14.8934) construction
  line L330 (42.3514, -14.8934) -> (42.3634, -14.8153) construction
  spline S96 degree 3 poles (42.3634, -14.8153) (42.3754, -14.7554) (42.3574, -14.6954) (42.3874, -14.6354) knots 10 10 10 10 11 11 11 11
  line L331 (42.3634, -14.8153) -> (42.3754, -14.7554) construction
  line L332 (42.3754, -14.7554) -> (42.3574, -14.6954) construction
  line L333 (42.3574, -14.6954) -> (42.3874, -14.6354) construction
  spline S97 degree 3 poles (42.3874, -14.6354) (42.4054, -14.5993) (42.4114, -14.6053) (42.4534, -14.5933) knots 11 11 11 11 12 12 12 12
  line L334 (42.3874, -14.6354) -> (42.4054, -14.5993) construction
  line L335 (42.4054, -14.5993) -> (42.4114, -14.6053) construction
  line L336 (42.4114, -14.6053) -> (42.4534, -14.5933) construction
  line L337 (42.4534, -14.5933) -> (42.5554, -14.5574)
  spline S98 degree 3 poles (42.5554, -14.5574) (42.6214, -14.5333) (42.6874, -14.5094) (42.7474, -14.4733) knots 13 13 13 13 14 14 14 14
  line L338 (42.5554, -14.5574) -> (42.6214, -14.5333) construction
  line L339 (42.6214, -14.5333) -> (42.6874, -14.5094) construction
  line L340 (42.6874, -14.5094) -> (42.7474, -14.4733) construction
  spline S99 degree 3 poles (42.7474, -14.4733) (42.8374, -14.4194) (42.9213, -14.3534) (42.9993, -14.2874) knots 14 14 14 14 15 15 15 15
  line L341 (42.7474, -14.4733) -> (42.8374, -14.4194) construction
  line L342 (42.8374, -14.4194) -> (42.9213, -14.3534) construction
  line L343 (42.9213, -14.3534) -> (42.9993, -14.2874) construction
  spline S100 degree 3 poles (42.9993, -14.2874) (43.1853, -14.1314) (43.3833, -13.9454) (43.4613, -13.7114) knots 15 15 15 15 16 16 16 16
  line L344 (42.9993, -14.2874) -> (43.1853, -14.1314) construction
  line L345 (43.1853, -14.1314) -> (43.3833, -13.9454) construction
  line L346 (43.3833, -13.9454) -> (43.4613, -13.7114) construction
  spline S101 degree 3 poles (43.4613, -13.7114) (43.5033, -13.5794) (43.5094, -13.4354) (43.4253, -13.3214) knots 16 16 16 16 17 17 17 17
  line L347 (43.4613, -13.7114) -> (43.5033, -13.5794) construction
  line L348 (43.5033, -13.5794) -> (43.5094, -13.4354) construction
  line L349 (43.5094, -13.4354) -> (43.4253, -13.3214) construction
  spline S102 degree 3 poles (43.4253, -13.3214) (43.3474, -13.2194) (43.2154, -13.1654) (43.0954, -13.1414) knots 17 17 17 17 18 18 18 18
  line L350 (43.4253, -13.3214) -> (43.3474, -13.2194) construction
  line L351 (43.3474, -13.2194) -> (43.2154, -13.1654) construction
  line L352 (43.2154, -13.1654) -> (43.0954, -13.1414) construction
  spline S103 degree 3 poles (43.0954, -13.1414) (42.7714, -13.0814) (42.5253, -13.2674) (42.3394, -13.5134) knots 18 18 18 18 19 19 19 19
  line L353 (43.0954, -13.1414) -> (42.7714, -13.0814) construction
  line L354 (42.7714, -13.0814) -> (42.5253, -13.2674) construction
  line L355 (42.5253, -13.2674) -> (42.3394, -13.5134) construction
  spline S104 degree 3 poles (42.3394, -13.5134) (42.202, -13.6833) (42.0892, -13.8773) (42.0036, -14.082) knots 19 19 19 19 20 20 20 20
  line L356 (42.3394, -13.5134) -> (42.202, -13.6833) construction
  line L357 (42.202, -13.6833) -> (42.0892, -13.8773) construction
  line L358 (42.0892, -13.8773) -> (42.0036, -14.082) construction
  spline S105 degree 3 poles (42.0036, -14.082) (41.9329, -14.1729) (41.8829, -14.304) (41.8234, -14.4013) knots 20 20 20 20 21 21 21 21
  line L359 (42.0036, -14.082) -> (41.9329, -14.1729) construction
  line L360 (41.9329, -14.1729) -> (41.8829, -14.304) construction
  line L361 (41.8829, -14.304) -> (41.8234, -14.4013) construction
  spline S106 degree 3 poles (41.8234, -14.4013) (41.7214, -14.5754) (41.6194, -14.7433) (41.5114, -14.9113) knots 21 21 21 21 22 22 22 22
  line L362 (41.8234, -14.4013) -> (41.7214, -14.5754) construction
  line L363 (41.7214, -14.5754) -> (41.6194, -14.7433) construction
  line L364 (41.6194, -14.7433) -> (41.5114, -14.9113) construction
  spline S107 degree 3 poles (41.5114, -14.9113) (41.3074, -15.2353) (41.1034, -15.5653) (40.8574, -15.8593) knots 22 22 22 22 23 23 23 23
  line L365 (41.5114, -14.9113) -> (41.3074, -15.2353) construction
  line L366 (41.3074, -15.2353) -> (41.1034, -15.5653) construction
  line L367 (41.1034, -15.5653) -> (40.8574, -15.8593) construction
  spline S108 degree 3 poles (40.8574, -15.8593) (40.7554, -15.9853) (40.5394, -16.2913) (40.3354, -16.2673) knots 23 23 23 23 24 24 24 24
  line L368 (40.8574, -15.8593) -> (40.7554, -15.9853) construction
  line L369 (40.7554, -15.9853) -> (40.5394, -16.2913) construction
  line L370 (40.5394, -16.2913) -> (40.3354, -16.2673) construction
  spline S109 degree 3 poles (40.3354, -16.2673) (40.1854, -16.2433) (40.1854, -15.9853) (40.1854, -15.8713) (40.1854, -15.7753) (40.1914, -15.6793) (40.2035, -15.5893) knots 24 24 24 24 25 25 25 26 26 26 26
  line L371 (40.3354, -16.2673) -> (40.1854, -16.2433) construction
  line L372 (40.1854, -16.2433) -> (40.1854, -15.9853) construction
  line L373 (40.1854, -15.9853) -> (40.1854, -15.8713) construction
  line L374 (40.1854, -15.8713) -> (40.1854, -15.7753) construction
  line L375 (40.1854, -15.7753) -> (40.1914, -15.6793) construction
  line L376 (40.1914, -15.6793) -> (40.2035, -15.5893) construction
  spline S110 degree 3 poles (40.2035, -15.5893) (40.2094, -15.5353) (40.2574, -15.3553) (40.2274, -15.3073) knots 26 26 26 26 27 27 27 27
  line L377 (40.2035, -15.5893) -> (40.2094, -15.5353) construction
  line L378 (40.2094, -15.5353) -> (40.2574, -15.3553) construction
  line L379 (40.2574, -15.3553) -> (40.2274, -15.3073) construction
  line L380 (40.2274, -15.3073) -> (40.1794, -15.4873)
  spline S111 degree 3 poles (40.1794, -15.4873) (40.1854, -15.4153) (40.1974, -15.3373) (40.2154, -15.2653) knots 28 28 28 28 29 29 29 29
  line L381 (40.1794, -15.4873) -> (40.1854, -15.4153) construction
  line L382 (40.1854, -15.4153) -> (40.1974, -15.3373) construction
  line L383 (40.1974, -15.3373) -> (40.2154, -15.2653) construction
  spline S112 degree 3 poles (40.2154, -15.2653) (40.2094, -15.2533) (40.2634, -15.0853) (40.2754, -15.0314) knots 29 29 29 29 30 30 30 30
  line L384 (40.2154, -15.2653) -> (40.2094, -15.2533) construction
  line L385 (40.2094, -15.2533) -> (40.2634, -15.0853) construction
  line L386 (40.2634, -15.0853) -> (40.2754, -15.0314) construction
  spline S113 degree 3 poles (40.2754, -15.0314) (40.3054, -14.9113) (40.3354, -14.7913) (40.3714, -14.6713) knots 30 30 30 30 31 31 31 31
  line L387 (40.2754, -15.0314) -> (40.3054, -14.9113) construction
  line L388 (40.3054, -14.9113) -> (40.3354, -14.7913) construction
  line L389 (40.3354, -14.7913) -> (40.3714, -14.6713) construction
  spline S114 degree 3 poles (40.3714, -14.6713) (40.4014, -14.5514) (40.4314, -14.4374) (40.4674, -14.3234) knots 31 31 31 31 32 32 32 32
  line L390 (40.3714, -14.6713) -> (40.4014, -14.5514) construction
  line L391 (40.4014, -14.5514) -> (40.4314, -14.4374) construction
  line L392 (40.4314, -14.4374) -> (40.4674, -14.3234) construction
  spline S115 degree 3 poles (40.4674, -14.3234) (40.4974, -14.2154) (40.5394, -14.1614) (40.6054, -14.0774) knots 32 32 32 32 33 33 33 33
  line L393 (40.4674, -14.3234) -> (40.4974, -14.2154) construction
  line L394 (40.4974, -14.2154) -> (40.5394, -14.1614) construction
  line L395 (40.5394, -14.1614) -> (40.6054, -14.0774) construction
  spline S116 degree 3 poles (40.6054, -14.0774) (40.8754, -13.7414) (41.1214, -13.3754) (41.3494, -13.0094) knots 33 33 33 33 34 34 34 34
  line L396 (40.6054, -14.0774) -> (40.8754, -13.7414) construction
  line L397 (40.8754, -13.7414) -> (41.1214, -13.3754) construction
  line L398 (41.1214, -13.3754) -> (41.3494, -13.0094) construction
  spline S117 degree 3 poles (41.3494, -13.0094) (41.4334, -12.8714) (41.4874, -12.7514) (41.5894, -12.6374) knots 34 34 34 34 35 35 35 35
  line L399 (41.3494, -13.0094) -> (41.4334, -12.8714) construction
  line L400 (41.4334, -12.8714) -> (41.4874, -12.7514) construction
  line L401 (41.4874, -12.7514) -> (41.5894, -12.6374) construction
  spline S118 degree 3 poles (41.5894, -12.6374) (41.7394, -12.4814) (41.8475, -12.2474) (41.9435, -12.0554) knots 35 35 35 35 36 36 36 36
  line L402 (41.5894, -12.6374) -> (41.7394, -12.4814) construction
  line L403 (41.7394, -12.4814) -> (41.8475, -12.2474) construction
  line L404 (41.8475, -12.2474) -> (41.9435, -12.0554) construction
  spline S119 degree 3 poles (41.9435, -12.0554) (42.1056, -11.7434) (42.3333, -11.3114) (42.2917, -10.9454) knots 36 36 36 36 37 37 37 37
  line L405 (41.9435, -12.0554) -> (42.1056, -11.7434) construction
  line L406 (42.1056, -11.7434) -> (42.3333, -11.3114) construction
  line L407 (42.3333, -11.3114) -> (42.2917, -10.9454) construction
  line L408 (42.2917, -10.9454) -> (42.2917, -10.9154)
  line L409 (42.2917, -10.9154) -> (42.2795, -10.9094)
  spline S120 degree 3 poles (42.2795, -10.9094) (42.2435, -10.6754) (42.0245, -10.3994) (41.7605, -10.4834) knots 39 39 39 39 40 40 40 40
  line L410 (42.2795, -10.9094) -> (42.2435, -10.6754) construction
  line L411 (42.2435, -10.6754) -> (42.0245, -10.3994) construction
  line L412 (42.0245, -10.3994) -> (41.7605, -10.4834) construction
  spline S121 degree 3 poles (41.7605, -10.4834) (41.6225, -10.5254) (41.519, -10.6694) (41.4349, -10.7714) knots 40 40 40 40 41 41 41 41
  line L413 (41.7605, -10.4834) -> (41.6225, -10.5254) construction
  line L414 (41.6225, -10.5254) -> (41.519, -10.6694) construction
  line L415 (41.519, -10.6694) -> (41.4349, -10.7714) construction
  line L416 (41.4349, -10.7714) -> (41.2962, -10.9574)
  spline S122 degree 3 poles (41.2962, -10.9574) (41.2662, -10.9934) (41.2238, -11.0834) (41.1938, -11.1314) knots 42 42 42 42 43 43 43 43
  line L417 (41.2962, -10.9574) -> (41.2662, -10.9934) construction
  line L418 (41.2662, -10.9934) -> (41.2238, -11.0834) construction
  line L419 (41.2238, -11.0834) -> (41.1938, -11.1314) construction
  line L420 (41.1938, -11.1314) -> (41.1996, -11.1254)
  line L421 (41.1996, -11.1254) -> (41.0075, -11.4554)
  line L422 (41.0075, -11.4554) -> (41.0555, -11.3534)
  spline S123 degree 3 poles (41.0555, -11.3534) (41.0255, -11.3474) (40.8935, -11.6054) (40.8754, -11.6354) knots 46 46 46 46 47 47 47 47
  line L423 (41.0555, -11.3534) -> (41.0255, -11.3474) construction
  line L424 (41.0255, -11.3474) -> (40.8935, -11.6054) construction
  line L425 (40.8935, -11.6054) -> (40.8754, -11.6354) construction
  spline S124 degree 3 poles (40.8754, -11.6354) (40.8094, -11.7494) (40.7494, -11.8634) (40.6954, -11.9774) knots 47 47 47 47 48 48 48 48
  line L426 (40.8754, -11.6354) -> (40.8094, -11.7494) construction
  line L427 (40.8094, -11.7494) -> (40.7494, -11.8634) construction
  line L428 (40.7494, -11.8634) -> (40.6954, -11.9774) construction
  spline S125 degree 3 poles (40.6954, -11.9774) (40.5754, -12.2174) (40.4554, -12.4634) (40.3774, -12.7214) knots 48 48 48 48 49 49 49 49
  line L429 (40.6954, -11.9774) -> (40.5754, -12.2174) construction
  line L430 (40.5754, -12.2174) -> (40.4554, -12.4634) construction
  line L431 (40.4554, -12.4634) -> (40.3774, -12.7214) construction
  spline S126 degree 3 poles (40.3774, -12.7214) (40.2934, -12.9794) (40.1974, -13.2314) (40.1074, -13.4894) knots 49 49 49 49 50 50 50 50
  line L432 (40.3774, -12.7214) -> (40.2934, -12.9794) construction
  line L433 (40.2934, -12.9794) -> (40.1974, -13.2314) construction
  line L434 (40.1974, -13.2314) -> (40.1074, -13.4894) construction
  spline S127 degree 3 poles (40.1074, -13.4894) (40.0594, -13.6274) (40.0114, -13.7714) (39.9694, -13.9094) knots 50 50 50 50 51 51 51 51
  line L435 (40.1074, -13.4894) -> (40.0594, -13.6274) construction
  line L436 (40.0594, -13.6274) -> (40.0114, -13.7714) construction
  line L437 (40.0114, -13.7714) -> (39.9694, -13.9094) construction
  spline S128 degree 3 poles (39.9694, -13.9094) (39.9526, -13.9626) (39.9254, -14.0316) (39.9029, -14.1023) knots 51 51 51 51 52 52 52 52
  line L438 (39.9694, -13.9094) -> (39.9526, -13.9626) construction
  line L439 (39.9526, -13.9626) -> (39.9254, -14.0316) construction
  line L440 (39.9254, -14.0316) -> (39.9029, -14.1023) construction
  spline S129 degree 3 poles (39.9029, -14.1023) (39.8236, -14.1637) (39.7421, -14.2598) (39.7234, -14.2753) knots 52 52 52 52 53 53 53 53
  line L441 (39.9029, -14.1023) -> (39.8236, -14.1637) construction
  line L442 (39.8236, -14.1637) -> (39.7421, -14.2598) construction
  line L443 (39.7421, -14.2598) -> (39.7234, -14.2753) construction
  spline S130 degree 3 poles (39.7234, -14.2753) (39.5494, -14.4673) (39.3875, -14.6773) (39.2314, -14.8873) knots 53 53 53 53 54 54 54 54
  line L444 (39.7234, -14.2753) -> (39.5494, -14.4673) construction
  line L445 (39.5494, -14.4673) -> (39.3875, -14.6773) construction
  line L446 (39.3875, -14.6773) -> (39.2314, -14.8873) construction
  spline S131 degree 3 poles (39.2314, -14.8873) (39.0754, -15.1034) (38.9255, -15.3193) (38.7634, -15.5353) knots 54 54 54 54 55 55 55 55
  line L447 (39.2314, -14.8873) -> (39.0754, -15.1034) construction
  line L448 (39.0754, -15.1034) -> (38.9255, -15.3193) construction
  line L449 (38.9255, -15.3193) -> (38.7634, -15.5353) construction
  spline S132 degree 3 poles (38.7634, -15.5353) (38.6855, -15.6433) (38.6075, -15.7453) (38.5175, -15.8413) knots 55 55 55 55 56 56 56 56
  line L450 (38.7634, -15.5353) -> (38.6855, -15.6433) construction
  line L451 (38.6855, -15.6433) -> (38.6075, -15.7453) construction
  line L452 (38.6075, -15.7453) -> (38.5175, -15.8413) construction
  spline S133 degree 3 poles (38.5175, -15.8413) (38.4875, -15.8773) (38.4154, -15.9793) (38.3615, -15.9793) (38.1514, -15.9793) (38.3134, -15.1333) (38.3374, -15.0013) knots 56 56 56 56 57 57 57 58 58 58 58
  line L453 (38.5175, -15.8413) -> (38.4875, -15.8773) construction
  line L454 (38.4875, -15.8773) -> (38.4154, -15.9793) construction
  line L455 (38.4154, -15.9793) -> (38.3615, -15.9793) construction